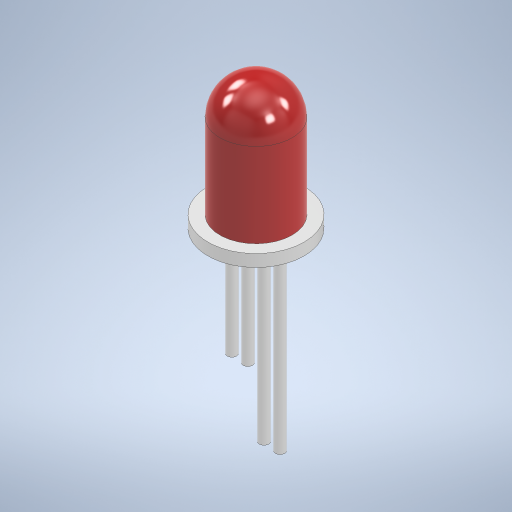
# Autodesk Inventor part: 8mm Through-Hole LED
Saved by Autodesk Inventor 2024.1 (Build 281209000, 209)
## iProperties
Created: 2023-12-30
Part Number: 8mm Through-Hole LED
Material: Aluminum
Document SubType Name: Modeling
Designer: ryanm
Density: 2.7 g/cm^3
Appearance: Satin
Author: ryanm
Autodesk Inventor part; units mm, degrees
ref_plane "YZ Plane" through (0, 0, 0) normal (1, 0, 0) x (0, 1, 0)
ref_plane "XZ Plane" through (0, 0, 0) normal (0, 1, 0) x (-1, 0, 0)
ref_plane "XY Plane" through (0, 0, 0) normal (0, 0, 1) x (1, 0, 0)
sketch "Sketch1" plane through (0, 0, 0) normal (0, 1, 0) x (-1, 0, 0)
  circle A0 centre (0, 0) radius 4
  dimension "d0" = 8
  constraints: 1 centre point, 1 coincident
  measures "d0" diameter of A0
extrude "Extrusion1" add sketch "Sketch1" along normal blind 1
sketch "Sketch2" plane through (0, 1, 0) normal (0, 1, 0) x (1, 0, 0)
  circle A0 centre (0, 0) radius 3
  dimension "d3" = 6
  constraints: 1 centre point, 1 coincident
  measures "d3" diameter of A0
extrude "Extrusion2" add sketch "Sketch2" along normal blind 10
fillet "Fillet1" radius 3 1 edges at (-3, 11, 0)
sketch "Sketch3" plane through (0, 0, 0) normal (0, -1, 0) x (1, 0, 0)
  circle A0 centre (-2, 0) radius 0.4
  circle A1 centre (-0.6667, 0) radius 0.4
  point P0 (0, 0)
  dimension "d7" = 0.8
  dimension "d8" = 0.6667
  dimension "d9" = 1.3333
  constraints: 2 centre point, 2 horizontal alignment, 1 equal radius
  measures "d7" diameter of A1
  measures "d8" distance of point (0, 0) A1.centre
  measures "d9" distance of A1.centre A0.centre
extrude "Extrusion3" add sketch "Sketch3" along normal blind 10
sketch "Sketch4" plane through (0, 0, 0) normal (0, -1, 0) x (1, 0, 0)
  circle A0 centre (0.6667, 0) radius 0.4
  circle A1 centre (2, 0) radius 0.4
  point P0 (0, 0)
  dimension "d12" = 0.8
  dimension "d13" = 0.8
  dimension "d14" = 0.6667
  dimension "d15" = 1.3333
  constraints: 2 centre point, 2 horizontal alignment
  measures "d12" diameter of A0
  measures "d13" diameter of A1
  measures "d14" distance of A0.centre point (0, 0)
  measures "d15" distance of A1.centre A0.centre
extrude "Extrusion4" add sketch "Sketch4" along normal blind 15
body "Solid1"
